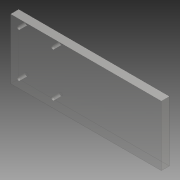
# Autodesk Inventor part: Spirulina_base
Saved by Autodesk Inventor 2016 (Build 200138000, 138)
## iProperties
Created: 2015-08-01
Part Number: Spirulina_base
Material: Generic
Document SubType Name: Modeling
Designer: Openlab
Density: 1 g/cm^3
Appearance: Polycarbonate - Clear
Author: Openlab
Autodesk Inventor part; units mm, degrees
ref_plane "YZ Plane" through (0, 0, 0) normal (1, 0, 0) x (0, 1, 0)
ref_plane "XZ Plane" through (0, 0, 0) normal (0, 1, 0) x (-1, 0, 0)
ref_plane "XY Plane" through (0, 0, 0) normal (0, 0, 1) x (1, 0, 0)
sketch "Sketch2" plane through (0, 0, 0) normal (0, 1, 0) x (-1, 0, 0)
  line L0 (0, 0) -> (150, 0)
  line L1 (150, 0) -> (150, -60)
  line L2 (150, -60) -> (0, -60)
  line L3 (0, -60) -> (0, 0)
  dimension "d0" = 150
  dimension "d1" = 60
  constraints: 8 end point, 2 parallel, 1 horizontal, 1 perpendicular
  measures "d0" distance of L1.end L2.end
  measures "d1" distance of L0.end L1.end
extrude "Extrusion1" add sketch "Sketch2" along normal blind 8
sketch "Sketch3" plane through (0, 8, 0) normal (0, 1, 0) x (1, 0, 0)
  line L0 (-105, 55) -> (-105, 5)
  line L1 (-110, 17.25) -> (-110, 25.75)
  line L2 (-110, 25.75) -> (-111, 25.75)
  line L3 (-111, 25.75) -> (-111, 17.25)
  line L4 (-111, 17.25) -> (-110, 17.25)
  line L5 (-111, 34.25) -> (-110, 34.25)
  line L6 (-110, 34.25) -> (-110, 42.75)
  line L7 (-110, 42.75) -> (-111, 42.75)
  line L8 (-111, 42.75) -> (-111, 34.25)
  line L9 (-105, 55) -> (-145, 55)
  line L10 (-145, 5) -> (-105, 5)
  line L11 (-125.0415, 30) -> (-130.864, 30) construction
  line L12 (-145, 5) -> (-145, 55)
  circle A0 centre (-108, 52) radius 1.5
  circle A1 centre (-142, 52) radius 1.5
  circle A2 centre (-108, 8) radius 1.5
  circle A3 centre (-142, 8) radius 1.5
  line L13 (-150, 60) -> (-150, 0) projected
  line L14 (0, 60) -> (-150, 60) projected
  point P0 (0, 0)
  point P1 (-109.5, 47)
  point P2 (-109.5, 30)
  point P3 (-109.5, 13)
  dimension "d34" = 8.5
  dimension "d35" = 1
  dimension "d36" = 5
  dimension "d37" = 17
  dimension "d38" = 17
  dimension "d39" = 4.25
  dimension "d40" = 4.25
  dimension "d41" = 4.5
  dimension "d42" = 40
  dimension "d43" = 50
  dimension "d44" = 3
  dimension "d45" = 3
  dimension "d46" = 3
  dimension "d47" = 3
  dimension "d48" = 3
  dimension "d49" = 5
  dimension "d50" = 5
  constraints: 26 end point, 6 perpendicular, 4 centre point, 4 coincident, 4 vertical alignment, 3 equal radius, 2 equal length, 2 horizontal, 2 horizontal alignment, 2 parallel, 2 point on line, 1 collinear, 1 vertical, 1 other
  measures "d34" distance of L7.end L5.start
  measures "d35" distance of L6.end L7.end
  measures "d36" distance between parallel lines of L0 L6
  measures "d37" distance of point (-109.5, 30) point (-109.5, 47)
  measures "d38" distance of point (-109.5, 13) point (-109.5, 30)
  measures "d39" distance from line of L7 point (-109.5, 47)
  measures "d40" distance from line of point (-109.5, 30) L2
  measures "d41" distance from line of L0 point (-109.5, 13)
  measures "d42" distance of L0.start L9.end
  measures "d43" distance of L0.start L0.end
  measures "d44" diameter of A0
  measures "d45" distance from line of L0 A0.centre
  measures "d46" distance from line of L9 A0.centre
  measures "d47" distance from line of L10 A3.centre
  measures "d48" distance from line of L12 A3.centre
  measures "d49" distance between parallel lines of L12 L13
  measures "d50" distance between parallel lines of L14 L9
hole "Hole1" at (-108, 8, -8) at (-108, 8, -52) at (-142, 8, -8) at (-142, 8, -52) direction (0, -1, 0) diameter 3 end through all
body "Solid1"
